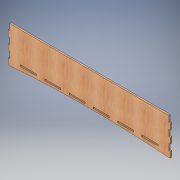
# Autodesk Inventor part: back
Saved by Autodesk Inventor 2016 (Build 200138000, 138)
## iProperties
Created: 2017-02-03
Part Number: back
Material: Wood (Birch)
Document SubType Name: Modeling
Designer: jwillauer
Density: 0.55 g/cm^3
Appearance: Birch - Natural Polished
Mass: 9122.01 g
Surface Area: 18390.4 cm^2
Volume: 16585.5 cm^3
Author: jwillauer
Autodesk Inventor part; units mm, degrees
ref_plane "YZ Plane" through (0, 0, 0) normal (1, 0, 0) x (0, 1, 0)
ref_plane "XZ Plane" through (0, 0, 0) normal (0, 1, 0) x (-1, 0, 0)
ref_plane "XY Plane" through (0, 0, 0) normal (0, 0, 1) x (1, 0, 0)
sketch "Sketch1" plane through (0, 0, 0) normal (0, 0, 1) x (1, 0, 0)
  line L0 (-998.1754, 340.1521) -> (1033.8246, 340.1521)
  line L1 (1033.8246, 340.1521) -> (1033.8246, -117.0479)
  line L2 (-998.1754, -117.0479) -> (-998.1754, 340.1521)
  arc A0 (995.7246, -117.0479) -> (-960.0754, -117.0479) centre (17.8246, -12647.7146) ccw
  line L3 (1033.8246, -117.0479) -> (995.7246, -117.0479)
  line L4 (-960.0754, -117.0479) -> (-998.1754, -117.0479)
  point P0 (0, 0)
  dimension "d0" = 2032
  dimension "d1" = 457.2
  constraints: 10 end point, 3 parallel, 2 point on circle, 1 centre point, 1 horizontal, 1 perpendicular
  measures "d0" distance of L0.start L0.end
  measures "d1" distance of L0.end L1.end
extrude "Extrusion1" add sketch "Sketch1" along normal blind 19.05
sketch "Sketch2" plane through (0, 0, 19.05) normal (0, 0, 1) x (1, 0, 0)
  line L0 (1033.8246, 340.1521) -> (-998.1754, 340.1521) projected
  line L1 (-998.1754, -117.0479) -> (-960.0754, -117.0479) projected
  line L2 (-998.1754, 340.1521) -> (-979.1254, 340.1521)
  line L3 (-979.1254, 340.1521) -> (-979.1254, -117.0479)
  line L4 (-979.1254, -117.0479) -> (-998.1754, -117.0479)
  line L5 (-998.1754, -117.0479) -> (-998.1754, 340.1521)
  line L6 (1033.8246, -117.0479) -> (1033.8246, 340.1521) projected
  line L7 (1033.8246, 340.1521) -> (1014.7746, 340.1521)
  line L8 (1014.7746, 340.1521) -> (1014.7746, -117.0479)
  line L9 (1014.7746, -117.0479) -> (1033.8246, -117.0479)
  line L10 (1033.8246, -117.0479) -> (1033.8246, 340.1521)
  line L11 (-998.1754, 340.1521) -> (-998.1754, -117.0479) projected
  line L12 (-998.1754, 263.9521) -> (-979.1254, 263.9521)
  line L13 (1014.7746, 263.9521) -> (1033.8246, 263.9521)
  line L14 (-998.1754, 187.7521) -> (-979.1254, 187.7521)
  line L15 (1014.7746, 187.7521) -> (1033.8246, 187.7521)
  line L16 (-998.1754, 111.5521) -> (-979.1254, 111.5521)
  line L17 (1014.7746, 111.5521) -> (1033.8246, 111.5521)
  line L18 (-998.1754, 35.3521) -> (-979.1254, 35.3521)
  line L19 (1014.7746, 35.3521) -> (1033.8246, 35.3521)
  line L20 (1033.8246, -40.8479) -> (1014.7746, -40.8479)
  line L21 (-979.1254, -40.8479) -> (-998.1754, -40.8479)
  point P0 (0, 0)
  dimension "d7" = 19.05
  dimension "d8" = 19.05
  constraints: 36 end point, 17 point on line, 12 perpendicular, 5 midpoint, 4 parallel, 2 horizontal
  measures "d7" distance between parallel lines of L3 L5
  measures "d8" distance between parallel lines of L6 L8
extrude "Extrusion2" cut sketch "Sketch2" against normal blind 19.05 contours L6 L13 L8 L0 | L3 L12 L5 L0 | L6 L17 L8 L15 | L3 L16 L5 L14 | L6 L20 L8 L19 | L3 L21 L5 L18
sketch "Sketch4" plane through (0, 0, 19.05) normal (0, 0, 1) x (1, 0, 0)
  line L0 (-845.7754, -40.8479) -> (-845.7754, -59.8979)
  line L1 (-998.1754, 111.5521) -> (-998.1754, 35.3521) projected
  line L2 (-642.5754, -40.8479) -> (-642.5754, -59.8979)
  line L3 (-540.9754, -40.8479) -> (-540.9754, -59.8979)
  line L4 (-337.7754, -40.8479) -> (-337.7754, -59.8979)
  line L5 (-236.1754, -40.8479) -> (-236.1754, -59.8979)
  line L6 (-32.9754, -40.8479) -> (-32.9754, -59.8979)
  line L7 (68.6246, -40.8479) -> (68.6246, -59.8267)
  line L8 (271.8246, -40.8479) -> (271.8246, -59.8267)
  line L9 (373.4246, -40.8479) -> (373.4246, -59.8979)
  line L10 (576.6246, -40.8479) -> (576.6246, -59.8979)
  line L11 (678.2246, -40.8479) -> (678.2246, -59.8979)
  line L12 (881.4246, -40.8479) -> (881.4246, -59.8979)
  arc A0 (995.7246, -117.0479) -> (-960.0754, -117.0479) centre (17.8246, -12647.7146) ccw projected
  line L13 (-998.1754, -40.8479) -> (-998.1754, -117.0479) projected
  line L14 (1014.7746, 340.1521) -> (-979.1254, 340.1521) projected
  line L15 (1014.7746, 340.1521) -> (1014.7746, 263.9521) projected
  line L16 (-979.1254, 340.1521) -> (1014.7746, 340.1521)
  line L17 (-845.7754, -40.8479) -> (-642.5754, -40.8479)
  line L18 (-845.7754, -59.8979) -> (-642.5754, -59.8979)
  line L19 (-540.9754, -59.8979) -> (-337.7754, -59.8979)
  line L20 (-540.9754, -40.8479) -> (-337.7754, -40.8479)
  line L21 (-236.1754, -40.8479) -> (-32.9754, -40.8479)
  line L22 (68.6246, -40.8479) -> (271.8246, -40.8479)
  line L23 (373.4246, -59.8979) -> (576.6246, -59.8979)
  line L24 (678.2246, -59.8979) -> (881.4246, -59.8979)
  line L25 (373.4246, -40.8479) -> (576.6246, -40.8479)
  line L26 (678.2246, -40.8479) -> (881.4246, -40.8479)
  line L27 (-236.1754, -59.8979) -> (-32.9754, -59.8979)
  line L28 (68.6246, -59.8267) -> (271.8246, -59.8267)
  point P0 (0, 0)
  dimension "d18" = 152.4
  dimension "d19" = 203.2
  dimension "d26" = 457.2
  dimension "d27" = 203.2
  dimension "d28" = 101.6
  dimension "d29" = 203.2
  dimension "d30" = 101.6
  dimension "d31" = 101.6
  dimension "d32" = 101.6
  dimension "d33" = 203.2
  dimension "d34" = 203.2
  dimension "d35" = 203.2
  constraints: 51 end point, 12 horizontal, 12 vertical, 1 perpendicular
  measures "d18" distance between parallel lines of L0 L1
  measures "d19" distance between parallel lines of L2 L0
  measures "d26" distance from line of L3.start L13
  measures "d27" distance of L3.end L4.end
  measures "d28" distance from line of L5.end L4
  measures "d29" distance of L5.start L6.start
  measures "d30" distance of L7.end L6.end
  measures "d31" distance from line of L9.end L8
  measures "d32" distance from line of L11 L10.end
  measures "d33" distance of L7.end L8.end
  measures "d34" distance of L9.end L10.end
  measures "d35" distance of L11.end L12.end
extrude "Extrusion4" cut sketch "Sketch4" against normal blind 25.4
body "Solid1"
